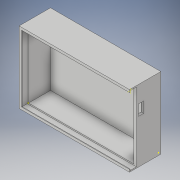
# Autodesk Inventor part: finalCase
Saved by Autodesk Inventor 2018.3 (Build 223284000, 284)
## iProperties
Created: 2019-04-19
Part Number: finalCase
Material: Generic
Document SubType Name: Modeling
Designer: Carlos Lopez
Density: 1 g/cm^3
Appearance: Default
Author: Carlos Lopez
Autodesk Inventor part; units mm, degrees
ref_plane "YZ Plane" through (0, 0, 0) normal (1, 0, 0) x (0, 1, 0)
ref_plane "XZ Plane" through (0, 0, 0) normal (0, 1, 0) x (-1, 0, 0)
ref_plane "XY Plane" through (0, 0, 0) normal (0, 0, 1) x (1, 0, 0)
sketch "Sketch1" plane through (0, 0, 0) normal (0, 0, 1) x (1, 0, 0)
  line L0 (0, 0) -> (83.9978, 0)
  line L1 (83.9978, 0) -> (83.9978, 52.9999)
  line L2 (83.9978, 52.9999) -> (0, 52.9999)
  line L3 (0, 52.9999) -> (0, 0)
  dimension "d0" = 83.9978
  dimension "d1" = 52.9999
  constraints: 8 end point, 2 parallel, 1 horizontal, 1 perpendicular
  measures "d0" distance of L2.end L1.end
  measures "d1" distance of L1.end L0.end
extrude "Extrusion1" add sketch "Sketch1" along normal blind 22.9997
shell "Shell1" thickness 1.9812 outward yes removed faces 1 at (55.9985, 17.6666, 22.9997)
sketch "Sketch2" plane through (85.979, -1.9812, -1.9812) normal (1, 0, 0) x (0, 0, -1)
  point P0 (-1.9812, 1.9812)
sketch "Sketch3" plane through (85.979, -1.9812, -1.9812) normal (1, 0, 0) x (0, 0, -1)
  line L0 (-13.7922, 43.5102) -> (-17.78, 43.5102)
  line L1 (-17.78, 43.5102) -> (-17.78, 35.0012)
  line L2 (-17.78, 35.0012) -> (-13.7922, 35.0012)
  line L3 (-13.7922, 35.0012) -> (-13.7922, 43.5102)
  point P0 (-1.9812, 1.9812)
  dimension "d5" = 3.9878
  dimension "d6" = 8.509
  constraints: 8 end point, 2 parallel, 1 horizontal, 1 perpendicular
  measures "d5" distance of L2.end L1.end
  measures "d6" distance of L1.end L0.end
extrude "Extrusion2" cut sketch "Sketch3" against normal blind 22.9997
sketch "Sketch4" plane through (85.979, -1.9812, -1.9812) normal (1, 0, 0) x (0, 0, -1)
  line L0 (-19.5072, 55.9816) -> (-24.5072, 55.9816)
  line L1 (-24.5072, 55.9816) -> (-24.5072, 0.9817)
  line L2 (-24.5072, 0.9817) -> (-19.5072, 0.9817)
  line L3 (-19.5072, 0.9817) -> (-19.5072, 55.9816)
  point P0 (-1.9812, 1.9812)
  dimension "d9" = 5
  dimension "d10" = 54.9999
  constraints: 8 end point, 2 parallel, 1 horizontal, 1 perpendicular
  measures "d9" distance of L2.end L1.end
  measures "d10" distance of L1.end L0.end
extrude "Extrusion3" cut sketch "Sketch4" against normal blind 87.0001
sketch "Sketch5" plane through (85.979, -0.9995, 17.526) normal (0, 0, 1) x (1, 0, 0)
  point P0 (-85.979, 0.9995)
sketch "Sketch6" plane through (85.979, -1.9812, -1.9812) normal (1, 0, 0) x (0, 0, -1)
  point P0 (-1.9812, 1.9812)
  point P1 (-24.5072, 55.9816)
sketch "Sketch7" plane through (0, 0, 22.9997) normal (0, 0, 1) x (1, 0, 0)
  line L0 (83.9978, 52.9999) -> (0, 52.9999) projected
  line L1 (85.979, -1.9812) -> (85.979, 54.9811) projected
  line L2 (83.9978, 52.9999) -> (85.979, 52.9999)
  line L3 (85.979, 52.9999) -> (85.979, 0)
  line L4 (85.979, 0) -> (83.9978, 0)
  line L5 (83.9978, 0) -> (83.9978, 52.9999)
  point P0 (0, 0)
  constraints: 8 end point, 2 parallel, 1 horizontal, 1 perpendicular, 1 point on line
extrude "Extrusion4" cut sketch "Sketch7" against normal blind 2.0066
body "Solid1"
